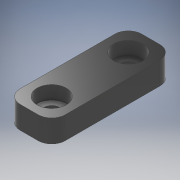
# Autodesk Inventor part: Belt Clamp Block
Saved by Autodesk Inventor 2020.2 (Build 242310000, 310)
## iProperties
Created: 2020-03-10
Part Number: Belt Clamp Block
Material: ABS Plastic
Document SubType Name: Modeling
Designer: Richard Hall
Density: 1.06 g/cm^3
Appearance: Satin - Black
Author: Richard Hall
Autodesk Inventor part; units mm, degrees
ref_plane "YZ Plane" through (0, 0, 0) normal (1, 0, 0) x (0, 1, 0)
ref_plane "XZ Plane" through (0, 0, 0) normal (0, 1, 0) x (-1, 0, 0)
ref_plane "XY Plane" through (0, 0, 0) normal (0, 0, 1) x (1, 0, 0)
sketch "Sketch1" plane through (0, 0, 0) normal (0, 1, 0) x (-1, 0, 0)
  line L0 (5, -13.5) -> (-5, -13.5)
  line L1 (-5, -13.5) -> (-5, 13.5)
  line L2 (-5, 13.5) -> (5, 13.5)
  line L3 (5, 13.5) -> (5, -13.5)
  line L4 (5, -13.5) -> (-5, 13.5) construction
  line L5 (-5, -13.5) -> (5, 13.5) construction
  circle A0 centre (0, -8.5) radius 3.25
  circle A1 centre (0, 8.5) radius 3.25
  circle A2 centre (0, 0) radius 1.5
  dimension "d0" = 17
  dimension "d1" = 6.5
  dimension "d2" = 6.5
  dimension "d3" = 3
  dimension "d4" = 5
  dimension "d5" = 5
  dimension "d6" = 5
  constraints: 12 end point, 3 centre point, 3 midpoint, 2 parallel, 2 vertical alignment, 1 coincident, 1 horizontal, 1 perpendicular
  measures "d0" distance of A1.centre A0.centre
  measures "d1" diameter of A0
  measures "d2" diameter of A1
  measures "d3" diameter of A2
  measures "d4" distance from line of A0.centre L3
  measures "d5" distance from line of L0 A0.centre
  measures "d6" distance from line of L2 A1.centre
extrude "Extrusion1" add sketch "Sketch1" along normal blind 5 contours L0 L1 L2 L3 | A0 | A1 | A2
sketch "Sketch2" plane through (0, 0, 0) normal (0, -1, 0) x (1, 0, 0)
  circle A0 centre (0, 0) radius 1.5
  dimension "d9" = 3
  constraints: 1 centre point, 1 coincident
  measures "d9" diameter of A0
extrude "Extrusion2" add sketch "Sketch2" along normal blind 1
sketch "Sketch3" plane through (0, 5, 0) normal (0, 1, 0) x (1, 0, 0)
  line L0 (-5, -13.5) -> (5, -13.5) projected
  line L1 (5, -13.5) -> (5, 13.5) projected
  line L2 (5, 13.5) -> (-5, 13.5) projected
  line L3 (-5, 13.5) -> (-5, -13.5) projected
  point P0 (0, 0)
  point P1 (0, 8.5)
  point P2 (0, -8.5)
  dimension "d12" = 8.5
  dimension "d13" = 8.5
  constraints: 2 vertical alignment
  measures "d12" distance of point (0, 0) point (0, 8.5)
  measures "d13" distance of point (0, -8.5) point (0, 0)
hole "Hole1" at (0, 5, -8.5) at (0, 5, 8.5) direction (0, -1, 0) diameter 3.6 depth 28.25 tip angle 118 counterbore diameter 6.5 counterbore depth 3 clearance for "Socket Head Cap Screw" size "M3" standard "Ansi Metric M Profile"
fillet "Fillet1" radius 3 4 edges at (5, 2.5, 13.5) (5, 2.5, -13.5) (-5, 2.5, -13.5) (-5, 2.5, 13.5)
sketch "Sketch4" plane through (0, 2, -8.5) normal (0, 1, 0) x (1, 0, 0)
  circle A0 centre (0, 0) radius 1.8 projected
  circle A1 centre (0, -17) radius 1.8 projected
  point P0 (0, -8.5)
extrude "Extrusion3" [suppressed]
equation "\"d13\" = d12"
body "Solid1"
